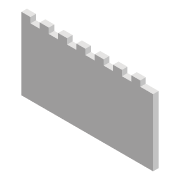
# Autodesk Inventor part: 00_Baseplate_Simmo_side7_v2
Saved by Autodesk Inventor 2022 (Build 260153000, 153)
## iProperties
Created: 2022-08-09
Part Number: 00_Baseplate_Simmo_side7_v2
Material: Generic
Document SubType Name: Modeling
Designer: wanghaoran
Density: 1 g/cm^3
Appearance: Default
Author: wanghaoran
Autodesk Inventor part; units mm, degrees
ref_plane "YZ Plane" through (0, 0, 0) normal (1, 0, 0) x (0, 1, 0)
ref_plane "XZ Plane" through (0, 0, 0) normal (0, 1, 0) x (-1, 0, 0)
ref_plane "XY Plane" through (0, 0, 0) normal (0, 0, 1) x (1, 0, 0)
sketch "Sketch1" plane through (0, 0, 0) normal (0, 0, 1) x (1, 0, 0)
  line L0 (-10, 0) -> (-10, 6) projected
  line L1 (133.8836, 0) -> (133.8836, 6) projected
  line L2 (133.8836, 6) -> (-10, 6)
  line L3 (-10, 6) -> (-10, -73)
  line L4 (-10, -73) -> (133.8836, -73)
  line L5 (133.8836, -73) -> (133.8836, 6)
  point P0 (0, 0)
  dimension "d0" = 79
  constraints: 8 end point, 2 parallel, 1 horizontal, 1 perpendicular
  measures "d0" distance of L3.end L2.end
extrude "Extrusion1" add sketch "Sketch1" along normal blind 6
sketch "Sketch2" plane through (0, 0, 6) normal (0, 0, 1) x (1, 0, 0)
  line L0 (110, 0) -> (110, 6) projected
  line L1 (100, 6) -> (100, 0) projected
  line L2 (133.8836, 6) -> (-10, 6) projected
  line L3 (110.1, 6) -> (99.9, 6)
  line L4 (99.9, 6) -> (99.9, 0)
  line L5 (99.9, 0) -> (110.1, 0)
  line L6 (110.1, 0) -> (110.1, 6)
  point P0 (0, 0)
  dimension "d3" = 10.2
  dimension "d4" = 6
  constraints: 8 end point, 2 parallel, 1 horizontal, 1 perpendicular, 1 point on line
  measures "d3" distance of L5.end L4.end
  measures "d4" distance of L4.end L3.end
extrude "Extrusion2" cut sketch "Sketch2" against normal blind 6
pattern_linear "Rectangular Pattern1" count 6 spacing 20 along (-1, 0, 0) of "Extrusion2"
sketch "Sketch3" plane through (0, 0, 6) normal (0, 0, 1) x (1, 0, 0)
  line L0 (120, 0) -> (133.8836, 0) projected
  line L1 (120, 6) -> (120, 0) projected
  line L2 (133.8836, 6) -> (110.1, 6) projected
  line L3 (133.8836, 0) -> (133.8836, 6) projected
  line L4 (120, 0) -> (119.9, 0)
  line L5 (119.9, 0) -> (119.9, 6)
  line L6 (119.9, 6) -> (120, 6)
  line L7 (120, 6) -> (120, 0)
  point P0 (0, 0)
  dimension "d10" = 0.1
  dimension "d11" = 6
  constraints: 8 end point, 2 parallel, 1 horizontal, 1 perpendicular
  measures "d10" distance of L5.end L6.end
  measures "d11" distance of L4.end L5.end
extrude "Extrusion3" cut sketch "Sketch3" against normal blind 6
body "Solid1"
